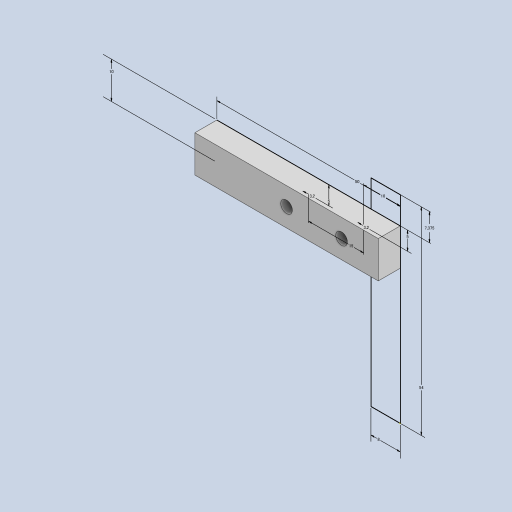
# Autodesk Inventor part: Part1
Saved by Autodesk Inventor 2023 (Build 270158000, 158)
## iProperties
Created: 2024-11-28
Part Number: Part1
Material: Generic
Document SubType Name: Modeling
Designer: kiyo
Density: 1 g/cm^3
Appearance: Default
Author: kiyo
Autodesk Inventor part; units mm, degrees
ref_plane "YZ Plane" through (0, 0, 0) normal (1, 0, 0) x (0, 1, 0)
ref_plane "XZ Plane" through (0, 0, 0) normal (0, 1, 0) x (-1, 0, 0)
ref_plane "XY Plane" through (0, 0, 0) normal (0, 0, 1) x (1, 0, 0)
sketch "スケッチ2" plane through (0, 0, 0) normal (1, 0, 0) x (0, 1, 0)
  line L0 (-50, 46.625) -> (0, 46.625)
  line L1 (0, 46.625) -> (0, 36.625)
  line L2 (0, 36.625) -> (-50, 36.625)
  line L3 (-50, 36.625) -> (-50, 46.625)
  line L4 (0, 36.625) -> (-8, 36.625)
  line L5 (-8, 36.625) -> (-8, 0)
  line L6 (-8, 0) -> (0, 0)
  line L7 (0, 0) -> (0, 36.625)
  circle A0 centre (-10, 41.625) radius 1.6
  circle A1 centre (-25, 41.625) radius 1.6
  line L8 (-8, 36.625) -> (0, 36.625)
  line L9 (0, 36.625) -> (0, 54)
  line L10 (0, 54) -> (-8, 54)
  line L11 (-8, 54) -> (-8, 36.625)
  dimension "d7" = 50
  dimension "d8" = 10
  dimension "d10" = 8
  dimension "d11" = 3.2
  dimension "d12" = 3.2
  dimension "d13" = 15
  dimension "d14" = 10
  dimension "d15" = 5
  dimension "d16" = 5
  dimension "d27" = 54
  dimension "d28" = 7.375
  constraints: 24 end point, 6 parallel, 3 horizontal, 3 perpendicular, 2 centre point, 1 coincident, 1 collinear
  measures "d7" distance of L0.start L0.end
  measures "d8" distance between parallel lines of L2 L0
  measures "d10" distance of L5.end L6.end
  measures "d11" diameter of A0
  measures "d12" diameter of A1
  measures "d13" distance of A0.centre A1.centre
  measures "d14" distance from line of L1 A0.centre
  measures "d15" distance from line of L0 A0.centre
  measures "d16" distance from line of L0 A1.centre
  measures "d27" distance between parallel lines of L6 L10
  measures "d28" distance between parallel lines of L0 L10
extrude "押し出し2" add sketch "スケッチ2" along normal blind 6 contours L0 L11 L2 L3 | L0 L1 L2 L11
